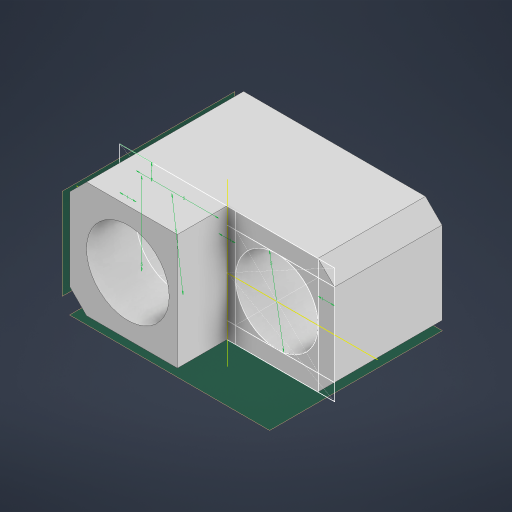
# Autodesk Inventor part: sensorholder_3
Saved by Autodesk Inventor 2023.5 (Build 275446000, 446)
## iProperties
Created: 2025-01-11
Part Number: sensorholder_3
Material: 一般
Document SubType Name: Modeling
Designer: IshiiLabHonda
Density: 1 g/cm^3
Appearance: 既定
Author: IshiiLabHonda
Autodesk Inventor part; units mm, degrees
ref_plane "YZ Plane" through (0, 0, 0) normal (1, 0, 0) x (0, 1, 0)
ref_plane "XZ Plane" through (0, 0, 0) normal (0, 1, 0) x (-1, 0, 0)
ref_plane "XY Plane" through (0, 0, 0) normal (0, 0, 1) x (1, 0, 0)
sketch "スケッチ1" plane through (0, 0, 0) normal (0, 0, 1) x (1, 0, 0)
  line L0 (-6.5, 3.5) -> (6.5, 3.5)
  line L1 (6.5, 3.5) -> (6.5, -3.5)
  line L2 (6.5, -3.5) -> (-6.5, -3.5)
  line L3 (-6.5, -3.5) -> (-6.5, 3.5)
  line L4 (-6.5, 3.5) -> (6.5, -3.5) construction
  line L5 (6.5, 3.5) -> (-6.5, -3.5) construction
  line L6 (5.5, 3.5) -> (5.5, -3.5)
  line L7 (0.5, 3.5) -> (0.5, -3.5)
  line L8 (-0.5, 3.5) -> (-0.5, -3.5)
  line L9 (-5.5, 3.5) -> (-5.5, -3.5)
  line L10 (0, -4.9) -> (0, 4.9) projected
  circle A0 centre (-3, 0) radius 2.5
  circle A1 centre (3, 0) radius 2.5
  line L11 (-6.5, -2.5) -> (6.5, -2.5)
  line L12 (-6.5, 2.5) -> (6.5, 2.5)
  line L13 (-9.1, 0) -> (9.1, 0) projected
  line L14 (-5.5, 2.5) -> (-0.5, -2.5) construction
  line L15 (-5.5, -2.5) -> (-0.5, 2.5) construction
  line L16 (5.5, 2.5) -> (0.5, -2.5) construction
  line L17 (5.5, -2.5) -> (0.5, 2.5) construction
  point P0 (0, 0)
  point P1 (0, 0)
  point P2 (3, 0)
  point P3 (-3, 0)
  point P4 (0, -3.5)
  point P5 (0, 3.5)
  dimension "d2" = 1
  dimension "d3" = 1
  dimension "d4" = 1
  dimension "d5" = 5
  dimension "d8" = 5
  dimension "d9" = 5
  dimension "d10" = 1
  dimension "d11" = 5
  constraints: 32 end point, 19 point on line, 7 parallel, 4 midpoint, 4 symmetric about line, 3 coincident, 2 centre point, 2 perpendicular, 1 horizontal, 2 other
  measures "d2" distance between parallel lines of L3 L9
  measures "d3" distance between parallel lines of L7 L8
  measures "d4" distance between parallel lines of L1 L6
  measures "d5" distance between parallel lines of L8 L9
  measures "d8" diameter of A0
  measures "d9" diameter of A1
  measures "d10" distance between parallel lines of L12 L0
  measures "d11" distance between parallel lines of L11 L12
extrude "押し出し1" add sketch "スケッチ1" against normal blind 6.5
extrude "押し出し2" add sketch "スケッチ1" along normal blind 3 contours L0 L9 L12 L3 | L0 L8 L12 L9 | L12 L9 L13 L3 | L0 L10 L12 L8 | L12 A0 L9 | L13 L9 L11 L3 | L12 L10 L13 L8 | L8 A0 L12 | A0 L11 L9 | L13 A0 | A0 L13 | L11 L9 L2 L3 | L13 L10 L11 L8 | L8 L11 A0 | L11 L8 L2 L9 | L11 L10 L2 L8
extrude "押し出し3" cut sketch "スケッチ1" along normal mid plane 20 contours L13 A0 | A0 L13 | L13 A1 | A1 L13
chamfer "面取り1" distance 1 angle 45 4 edges at (-6.5, 3.5, -1.75) (6.5, 3.5, -3.25) (6.5, -3.5, -3.25) (-6.5, -3.5, -1.75)
ref_plane "作業平面1" through (-5.5, -3.5, -6.5) normal (0, -1, 0) x (1, 0, 0)
sketch "スケッチ2" plane through (-5.5, -3.5, -6.5) normal (0, -1, 0) x (1, 0, 0)
  line L0 (0, 0) -> (0, 9.5) projected
  line L1 (11, 0) -> (0, 0) projected
  line L2 (11, 6.5) -> (11, 0) projected
  line L3 (5.5, 6.5) -> (11, 6.5) projected
  line L4 (5.5, 6.5) -> (5.5, 9.5) projected
  line L5 (0, 9.5) -> (5.5, 9.5) projected
  line L6 (0.5, 5.75) -> (10.5, 5.75)
  line L7 (10.5, 5.75) -> (10.5, 0.75)
  line L8 (10.5, 0.75) -> (0.5, 0.75)
  line L9 (0.5, 0.75) -> (0.5, 5.75)
  line L10 (0, 0) -> (0, 9.5) projected
  line L11 (11, 0) -> (12, 0) projected
  line L12 (0, 6.5) -> (11, 0) construction
  line L13 (5, 0) -> (0, 0) projected
  line L14 (12, 6.5) -> (11, 6.5) projected
  line L15 (0, 0) -> (11, 6.5) construction
  line L16 (12, 6.5) -> (-1, 6.5) projected
  line L17 (0.5, 5.75) -> (10.5, 0.75) construction
  line L18 (0.5, 0.75) -> (10.5, 5.75) construction
  point P0 (6.5, 6.5)
  point P1 (5.5, 3.25)
  dimension "d25" = 5
  dimension "d26" = 10
  constraints: 16 end point, 2 midpoint, 2 parallel, 2 point on line, 1 horizontal, 1 perpendicular
  measures "d25" distance between parallel lines of L6 L8
  measures "d26" distance between parallel lines of L7 L9
extrude "押し出し4" add sketch "スケッチ2" along normal blind 0.1 contours L6 L7 L8 L9
ref_plane "作業平面2" through (-6.5, -2.5, 3) normal (-1, 0, 0) x (0, 0, 1)
